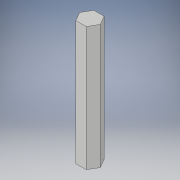
# Autodesk Inventor part: 3in hex shaft
Saved by Autodesk Inventor 2018 (Build 220112000, 112)
## iProperties
Created: 2018-01-18
Part Number: 3in hex shaft
Material: Generic
Document SubType Name: Modeling
Designer: maste
Density: 1 g/cm^3
Appearance: Default
Author: maste
Autodesk Inventor part; units mm, degrees
ref_plane "YZ Plane" through (0, 0, 0) normal (1, 0, 0) x (0, 1, 0)
ref_plane "XZ Plane" through (0, 0, 0) normal (0, 1, 0) x (-1, 0, 0)
ref_plane "XY Plane" through (0, 0, 0) normal (0, 0, 1) x (1, 0, 0)
sketch "Sketch1" plane through (0, 0, 0) normal (0, 1, 0) x (-1, 0, 0)
  line L0 (-7.3914, 0) -> (-3.6957, 6.4011)
  line L1 (-3.6957, 6.4011) -> (3.6957, 6.4011)
  line L2 (3.6957, 6.4011) -> (7.3914, 0)
  line L3 (7.3914, 0) -> (3.6957, -6.4011)
  line L4 (3.6957, -6.4011) -> (-3.6957, -6.4011)
  line L5 (-3.6957, -6.4011) -> (-7.3914, 0)
  point P0 (0, 0)
  point P1 (0, 0)
  dimension "d0" = 14.7828
  constraints: 12 end point, 1 coincident, 13 other
  measures "d0" distance of L0.start L2.end
extrude "Extrusion1" add sketch "Sketch1" along normal blind 88.9
body "Solid1"
